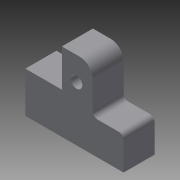
# Autodesk Inventor part: other side roller axle holder
Saved by Autodesk Inventor 2015 (Build 190159000, 159)
## iProperties
Created: 2014-09-20
Part Number: other side roller axle holder
Material: Generic
Document SubType Name: Modeling
Designer: jesse
Density: 1 g/cm^3
Appearance: Default
Author: jesse
Autodesk Inventor part; units mm, degrees
ref_plane "YZ Plane" through (0, 0, 0) normal (1, 0, 0) x (0, 1, 0)
ref_plane "XZ Plane" through (0, 0, 0) normal (0, 1, 0) x (-1, 0, 0)
ref_plane "XY Plane" through (0, 0, 0) normal (0, 0, 1) x (1, 0, 0)
ref_plane "FRONT" through (0, 0, 0) normal (0, 0, 1) x (1, 0, 0)
ref_plane "TOP" through (0, 0, 0) normal (0, 1, 0) x (-1, 0, 0)
ref_plane "RIGHT" through (0, 0, 0) normal (1, 0, 0) x (0, 1, 0)
ref_plane "Work Plane6" through (36, -22.5, -6.35) normal (0, 0, -1) x (-1, 0, 0)
sketch "Sketch1" plane through (36, -22.5, -6.35) normal (0, 0, -1) x (-1, 0, 0)
  line L0 (56.9176, 0) -> (29.4132, 0)
  line L1 (56.9176, 0) -> (29.4132, 0)
  line L2 (29.4132, 0) -> (29.4132, 32.1053)
  line L3 (41.9794, 32.1053) -> (41.9794, 16.7597)
  line L4 (29.4132, 32.1053) -> (41.9794, 32.1053)
  line L5 (41.9794, 16.7597) -> (56.9176, 16.7597)
  line L6 (56.9176, 16.7597) -> (56.9176, 0)
  point P0 (36, 22.5)
  point P1 (0, 0)
  constraints: 14 end point, 3 vertical, 2 perpendicular, 1 horizontal
extrude "Extrusion1" add sketch "Sketch1" along normal blind 12.7
ref_plane "Work Plane5" through (36, -22.5, -19.05) normal (0, 0, -1) x (-1, 0, 0)
sketch "Sketch2" plane through (36, -22.5, -19.05) normal (0, 0, -1) x (-1, 0, 0)
  circle A0 centre (36, 22.5) radius 3.1
  dimension "d2" = 6.2
  constraints: 1 centre point, 1 coincident
  measures "d2" diameter of A0
extrude "Extrusion2" cut sketch "Sketch2" against normal through all
ref_plane "Work Plane8" through (6.5868, -22.5, -6.35) normal (1, 0, 0) x (0, 0, -1)
sketch "Sketch3" plane through (6.5868, -22.5, -6.35) normal (1, 0, 0) x (0, 0, -1)
  line L0 (0, 32.1053) -> (0, 0) projected
  line L1 (0, 13.4651) -> (12.7, 13.4651)
  line L2 (12.7, 13.4651) -> (12.7, 0)
  line L3 (12.7, 0) -> (0, 0)
  line L4 (0, 0) -> (0, 13.4651)
  point P0 (-6.35, 22.5)
  point P1 (0, 26.9303)
  constraints: 8 end point, 2 parallel, 1 horizontal, 1 perpendicular, 1 point on line
extrude "Extrusion3" add sketch "Sketch3" along normal blind 12.7
sketch "Sketch4" plane through (36, -22.5, -19.05) normal (0, 0, -1) x (-1, 0, 0)
  circle A0 centre (36, 22.5) radius 3.1 projected
  line L0 (29.4132, 32.1053) -> (29.4132, 13.4651) projected
  line L1 (56.9176, 0) -> (16.7132, 0) projected
  line L2 (56.9176, 0) -> (56.9176, 16.7597) projected
  line L3 (56.9176, 16.7597) -> (41.9794, 16.7597) projected
  line L4 (41.9794, 16.7597) -> (41.9794, 32.1053) projected
  line L5 (41.9794, 32.1053) -> (29.4132, 32.1053) projected
  line L6 (16.7132, 0) -> (16.7132, 13.4651) projected
  line L7 (16.7132, 10.2251) -> (56.9176, 10.2251)
  line L8 (56.9176, 0) -> (56.9176, 16.7597) projected
  line L9 (41.9794, 16.7597) -> (41.9794, 10.2251)
  line L10 (29.4132, 13.4651) -> (29.4132, 10.2251)
  line L11 (29.4132, 13.4651) -> (16.7132, 13.4651)
  line L12 (16.7132, 13.4651) -> (16.7132, 10.2251)
  line L13 (41.9794, 16.7597) -> (56.9176, 16.7597)
  line L14 (56.9176, 16.7597) -> (56.9176, 10.2251)
  line L15 (29.4132, 13.4651) -> (16.7132, 13.4651)
  line L16 (16.7132, 13.4651) -> (16.7132, 10.2251)
  line L17 (16.7132, 10.2251) -> (29.4132, 10.2251)
  line L18 (29.4132, 10.2251) -> (29.4132, 13.4651)
  line L19 (41.9794, 16.7597) -> (56.9176, 16.7597)
  line L20 (56.9176, 16.7597) -> (56.9176, 10.2251)
  line L21 (56.9176, 10.2251) -> (41.9794, 10.2251)
  line L22 (41.9794, 10.2251) -> (41.9794, 16.7597)
  line L23 (29.4132, 13.4651) -> (16.7132, 13.4651) projected
  line L24 (16.7132, 0) -> (16.7132, 13.4651) projected
  constraints: 30 end point, 4 parallel, 4 perpendicular, 4 point on line, 3 horizontal, 2 collinear
extrude "Extrusion4" cut sketch "Sketch4" against normal through all contours L10 L7 L6 L11 | L3 L2 L7 L9
sketch "Sketch5" plane through (36, -22.5, -19.05) normal (0, 0, -1) x (-1, 0, 0)
  line L0 (56.9176, 0) -> (16.7132, 0) projected
  line L1 (56.9176, 0) -> (56.9176, 10.2251) projected
  line L2 (56.9176, 10.2251) -> (41.9794, 10.2251) projected
  line L3 (41.9794, 10.2251) -> (41.9794, 32.1053) projected
  line L4 (41.9794, 32.1053) -> (29.4132, 32.1053) projected
  line L5 (29.4132, 32.1053) -> (29.4132, 10.2251) projected
  circle A0 centre (36, 22.5) radius 3.1 projected
  line L6 (29.4132, 32.1053) -> (29.4132, 10.2251) projected
  line L7 (29.4132, 28.1591) -> (41.9794, 28.1591)
  line L8 (41.9794, 28.1591) -> (41.9794, 32.1053)
  line L9 (41.9794, 32.1053) -> (29.4132, 32.1053)
  line L10 (29.4132, 32.1053) -> (29.4132, 28.1591)
  line L11 (29.4132, 10.2251) -> (16.7132, 10.2251) projected
  line L12 (16.7132, 0) -> (16.7132, 10.2251) projected
  constraints: 8 end point, 2 parallel, 1 horizontal, 1 perpendicular, 1 point on line
extrude "Extrusion5" cut sketch "Sketch5" against normal through all contours L7 L5 L4 L3
fillet "Fillet4" radius 2 4 edges at (-5.9794, 5.6591, -12.7) (-5.9794, -12.2749, -12.7) (6.5868, 5.6591, -12.7) (-20.9176, -12.2749, -12.7)
ref_plane "Work Plane9" through (8.5868, -12.2749, -19.05) normal (0, 1, 0) x (1, 0, 0)
sketch "Sketch6" plane through (8.5868, -12.2749, -19.05) normal (0, 1, 0) x (1, 0, 0)
  line L0 (-2, 0) -> (10.7, 0) projected
  line L1 (10.7, -12.7) -> (-2, -12.7) projected
  line L2 (8.7, -6.35) -> (0, -6.35) construction
  line L3 (0, -12.7) -> (0, 0) construction
  line L4 (-29.5044, 0) -> (10.7, 0) construction
  line L5 (4.35, 0) -> (4.35, -12.7) construction
  line L6 (-29.5044, -12.7) -> (10.7, -12.7) construction
  circle A0 centre (4.35, -6.35) radius 1.7859
  line L7 (10.7, 0) -> (10.7, -12.7) projected
  line L8 (-2, 0) -> (-2, -12.7) projected
  point P0 (-8.5868, -19.05)
  point P1 (8.7, -12.7)
  point P2 (8.7, 0)
  dimension "d18" = 3.5719
  constraints: 4 end point, 2 midpoint, 2 point on line, 1 centre point, 1 perpendicular
  measures "d18" diameter of A0
extrude "Extrusion6" cut sketch "Sketch6" against normal through all contours A0
sketch "Sketch7" plane through (-18.9176, -12.2749, -19.05) normal (0, 1, 0) x (1, 0, 0)
  line L0 (0, -12.7) -> (0, 0) projected
  line L1 (10.9382, -12.7) -> (0, -12.7) projected
  line L2 (10.9382, 0) -> (10.9382, -12.7) projected
  line L3 (0, 0) -> (10.9382, 0) projected
  line L4 (5.4691, -12.7) -> (5.4691, 0) construction
  line L5 (-2, 0) -> (38.2044, 0) construction
  line L6 (10.9382, 0) -> (10.9382, -12.7) construction
  line L7 (10.9382, -6.35) -> (0, -6.35) construction
  circle A0 centre (5.4691, -6.35) radius 1.7859
  point P0 (18.9176, -19.05)
  point P1 (25.5044, 0)
  dimension "d21" = 3.5719
  constraints: 4 end point, 4 midpoint, 1 centre point, 1 perpendicular, 1 point on line
  measures "d21" diameter of A0
extrude "Extrusion7" cut sketch "Sketch7" against normal through all contours A0
